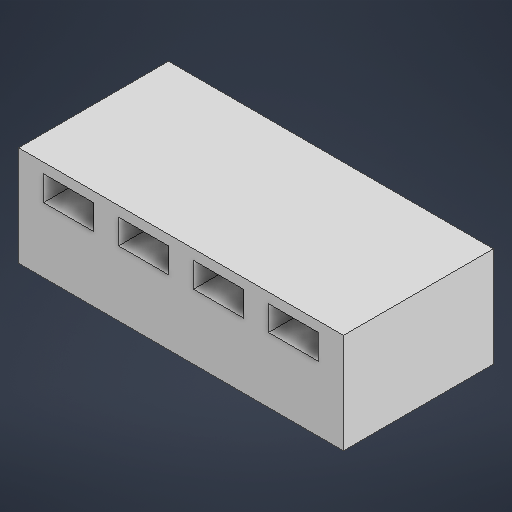
# Autodesk Inventor part: Relay
Saved by Autodesk Inventor 2026.2 (Build 302298000, 298)
## iProperties
Created: 2026-01-21
Part Number: Relay
Material: Generic
Document SubType Name: Modeling
Designer: User
Density: 1 g/cm^3
Appearance: Default
Author: User
Autodesk Inventor part; units mm, degrees
ref_plane "YZ Plane" through (0, 0, 0) normal (1, 0, 0) x (0, 1, 0)
ref_plane "XZ Plane" through (0, 0, 0) normal (0, 1, 0) x (-1, 0, 0)
sketch "Sketch1" plane through (0, 0, 0) normal (0, 1, 0) x (-1, 0, 0)
  line L0 (0, 0) -> (65, 0)
  line L1 (65, 0) -> (65, -30)
  line L2 (65, -30) -> (0, -30)
  line L3 (0, -30) -> (0, 0)
  dimension "d0" = 65
  dimension "d1" = 30
  constraints: 8 end point, 2 parallel, 1 horizontal, 1 perpendicular
  measures "d0" distance of L1.end L2.end
  measures "d1" distance of L0.end L1.end
extrude "Extrusion1" add sketch "Sketch1" along normal blind 20
sketch "Sketch2" plane through (-65, 0, 0) normal (0, 0, 1) x (1, 0, 0)
  line L0 (5, 18) -> (15, 18)
  line L1 (15, 18) -> (15, 13)
  line L2 (15, 13) -> (5, 13)
  line L3 (5, 13) -> (5, 18)
  line L4 (0, 0) -> (65, 0) projected
  line L5 (30, 18) -> (30, 13)
  line L6 (30, 13) -> (20, 13)
  line L7 (20, 13) -> (20, 18)
  line L8 (20, 18) -> (30, 18)
  line L9 (45, 18) -> (45, 13)
  line L10 (45, 13) -> (35, 13)
  line L11 (35, 13) -> (35, 18)
  line L12 (35, 18) -> (45, 18)
  line L13 (60, 18) -> (60, 13)
  line L14 (60, 13) -> (50, 13)
  line L15 (50, 13) -> (50, 18)
  line L16 (50, 18) -> (60, 18)
  dimension "d4" = 10
  dimension "d5" = 5
  dimension "d6" = 13
  dimension "d7" = 5
  dimension "d10" = 15
  constraints: 32 end point, 2 horizontal, 2 parallel, 1 perpendicular, 24 other
  measures "d4" distance of L0.start L0.end
  measures "d5" distance of L2.end L0.start
  measures "d6" distance between parallel lines of L4 L2
  measures "d7" distance from line of L4.start L3
  measures "d10" distance of L0.end L5.start
extrude "Extrusion2" cut sketch "Sketch2" against normal blind 10
ref_plane "Work Plane1" through (-65, 0, -15) normal (0, 0, 1) x (1, 0, 0)
mirror "Mirror1" about plane through (-65, 0, -15) normal (0, 0, 1) of "Extrusion2"
body "Solid1"
